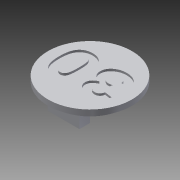
# Autodesk Inventor part: Inside
Saved by Autodesk Inventor 2014 (Build 180170000, 170)
## iProperties
Created: 2017-08-29
Part Number: Inside
Material: Generic
Document SubType Name: Modeling
Designer: resaj
Density: 1 g/cm^3
Appearance: White
Author: resaj
Autodesk Inventor part; units mm, degrees
ref_plane "YZ Plane" through (0, 0, 0) normal (1, 0, 0) x (0, 1, 0)
ref_plane "XZ Plane" through (0, 0, 0) normal (0, 1, 0) x (-1, 0, 0)
sketch "Sketch1" plane through (0, 0, 0) normal (0, 1, 0) x (-1, 0, 0)
  circle A0 centre (0, 0) radius 19.9
  dimension "d0" = 39.8
  constraints: 1 centre point, 1 coincident
  measures "d0" diameter of A0
extrude "Extrusion1" add sketch "Sketch1" along normal blind 2.6
sketch "Sketch2" plane through (0, 0, 0) normal (0, -1, 0) x (1, 0, 0)
  circle A0 centre (0, 0) radius 19.9 projected
  circle A1 centre (0, 0) radius 17.4
  dimension "d3" = 34.8
  constraints: 1 centre point, 1 coincident
  measures "d3" diameter of A1
extrude "Extrusion2" add sketch "Sketch2" along normal blind 2 contours A1
sketch "Sketch3" plane through (0, -2, 0) normal (0, -1, 0) x (1, 0, 0)
  circle A0 centre (0, 0) radius 17.4 projected
  line L0 (0, 0) -> (0, 17.4) construction
  line L1 (0, 0) -> (17.4, 0) construction
  line L2 (0, 12.5) -> (7.5, 12.5)
  line L3 (7.5, 12.5) -> (7.5, 7.5)
  line L4 (7.5, 7.5) -> (0, 7.5)
  line L5 (0, 12.5) -> (-7.5, 12.5)
  line L6 (-7.5, 12.5) -> (-7.5, 7.5)
  line L7 (-7.5, 7.5) -> (0, 7.5)
  line L8 (0, -12.5) -> (7.5, -12.5)
  line L9 (7.5, -12.5) -> (7.5, -7.5)
  line L10 (7.5, -7.5) -> (0, -7.5)
  line L11 (-7.5, -7.5) -> (0, -7.5)
  line L12 (-7.5, -12.5) -> (-7.5, -7.5)
  line L13 (0, -12.5) -> (-7.5, -12.5)
  dimension "d6" = 15
  dimension "d7" = 5
  dimension "d8" = 15
  constraints: 28 end point, 8 symmetric about line, 2 perpendicular, 2 point on circle, 2 point on line, 1 parallel, 1 vertical
  measures "d6" distance between parallel lines of L3 L6
  measures "d7" distance of L2.end L3.end
  measures "d8" distance between parallel lines of L10 L4
extrude "Extrusion3" add sketch "Sketch3" along normal blind 7.5 contours L2 L3 L4 L7 L6 L5 | L13 L12 L11 L10 L9 L8
ref_plane "Work Plane1" through (7.5, -9.5, 10) normal (0, 0, 1) x (1, 0, 0)
sketch "Sketch4" plane through (7.5, -2, -12.5) normal (0, 0, -1) x (-1, 0, 0)
  line L0 (0, 0) -> (15, 0) projected
  line L1 (0, 0) -> (0, -7.5) projected
  line L2 (15, -7.5) -> (0, -7.5) projected
  line L3 (15, 0) -> (15, -7.5) projected
  line L4 (2.35, 0) -> (2.35, -5.15)
  line L5 (2.35, -5.15) -> (12.65, -5.15)
  line L6 (12.65, -5.15) -> (12.65, 0)
  line L7 (2.35, -5.15) -> (0, -5.15) construction
  line L8 (2.35, -5.15) -> (2.35, -7.5) construction
  line L9 (12.65, -5.15) -> (15, -5.15) construction
  point P0 (7.5, 2)
  dimension "d11" = 10.3
  constraints: 12 end point, 7 perpendicular, 5 point on line, 1 parallel
  measures "d11" distance of L4.end L5.end
extrude "Extrusion4" cut sketch "Sketch4" against normal up to surface (22.5 mm away) contours L0 L6 L5 L4
sketch "Sketch5" plane through (0, 2.6, 0) normal (0, 1, 0) x (1, 0, 0)
  line L0 (15.5957, -8.6476) -> (-15.5957, -8.6476) construction
  line L1 (-15.5957, -8.6476) -> (-15.5957, 11.0665) construction
  line L2 (-15.5957, 11.0665) -> (15.5957, 11.0665) construction
  line L3 (15.5957, 11.0665) -> (15.5957, -8.6476) construction
  line L4 (14.5154, 4.6525) -> (10.6853, 4.2456)
  spline S0 degree 2 poles (10.6853, 4.2456) (10.531, 5.5083) (8.8755, 6.8551) (7.7391, 6.8551) knots 0 0 0 1 2 2 2
  spline S1 degree 2 poles (7.7391, 6.8551) (6.5185, 6.8551) (4.8209, 5.2558) (4.8209, 3.8528) knots 0 0 0 1 2 2 2
  spline S2 degree 2 poles (4.8209, 3.8528) (4.8209, 2.548) (6.4483, 1.0469) (7.6128, 1.0469) knots 0 0 0 1 2 2 2
  spline S3 degree 2 poles (7.6128, 1.0469) (8.3704, 1.0469) (9.4226, 1.2994) knots 0 0 0 1 1 1
  line L5 (9.4226, 1.2994) -> (8.9877, -1.5065)
  spline S4 degree 2 poles (8.9877, -1.5065) (7.4444, -1.4785) (6.5465, -2.0958) knots 0 0 0 1 1 1
  spline S5 degree 2 poles (6.5465, -2.0958) (5.6627, -2.7131) (5.6627, -3.8214) knots 0 0 0 1 1 1
  spline S6 degree 2 poles (5.6627, -3.8214) (5.6627, -4.7614) (6.9534, -5.8136) (7.9495, -5.8136) knots 0 0 0 1 2 2 2
  spline S7 degree 2 poles (7.9495, -5.8136) (8.9596, -5.8136) (10.4328, -4.593) (10.573, -3.4005) knots 0 0 0 1 2 2 2
  line L6 (10.573, -3.4005) -> (14.2348, -3.9477)
  spline S8 degree 2 poles (14.2348, -3.9477) (13.6596, -6.4169) (10.3486, -8.6476) (7.8373, -8.6476) knots 0 0 0 1 2 2 2
  spline S9 degree 2 poles (7.8373, -8.6476) (5.0033, -8.6476) (1.6783, -5.7715) (1.6783, -4.0318) knots 0 0 0 1 2 2 2
  spline S10 degree 2 poles (1.6783, -4.0318) (1.6783, -2.8534) (3.1654, -0.9594) (4.6666, -0.2579) knots 0 0 0 1 2 2 2
  spline S11 degree 2 poles (4.6666, -0.2579) (2.9269, 0.0788) (0.7523, 2.3376) (0.7523, 4.0212) knots 0 0 0 1 2 2 2
  spline S12 degree 2 poles (0.7523, 4.0212) (0.7523, 6.4904) (4.863, 9.7172) (7.711, 9.7172) knots 0 0 0 1 2 2 2
  spline S13 degree 2 poles (7.711, 9.7172) (10.4328, 9.7172) (14.2067, 6.9954) (14.5154, 4.6525) knots 0 0 0 1 2 2 2
  spline S14 degree 2 poles (-8.395, -8.6476) (-11.3973, -8.6476) (-15.1152, -4.565) (-15.1152, 0.5418) knots 0 0 0 1 2 2 2
  spline S15 degree 2 poles (-15.1152, 0.5418) (-15.1152, 5.6346) (-11.3973, 9.7172) (-8.409, 9.7172) knots 0 0 0 1 2 2 2
  spline S16 degree 2 poles (-8.409, 9.7172) (-5.4067, 9.7172) (-1.6888, 5.6626) (-1.6888, 0.4997) knots 0 0 0 1 2 2 2
  spline S17 degree 2 poles (-1.6888, 0.4997) (-1.6888, -4.565) (-5.4067, -8.6476) (-8.395, -8.6476) knots 0 0 0 1 2 2 2
  spline S18 degree 2 poles (-8.395, -5.7855) (-7.2165, -5.7855) (-5.8276, -3.5829) (-5.8276, 0.5418) knots 0 0 0 1 2 2 2
  spline S19 degree 2 poles (-5.8276, 0.5418) (-5.8276, 4.6665) (-7.2165, 6.8551) (-8.395, 6.8551) knots 0 0 0 1 2 2 2
  spline S20 degree 2 poles (-8.395, 6.8551) (-9.5735, 6.8551) (-10.9484, 4.6525) (-10.9484, 0.5418) knots 0 0 0 1 2 2 2
  spline S21 degree 2 poles (-10.9484, 0.5418) (-10.9484, -3.5829) (-9.5735, -5.7855) (-8.395, -5.7855) knots 0 0 0 1 2 2 2
  constraints: 2 other
extrude "Extrusion5" cut sketch "Sketch5" against normal blind 1
body "Solid1"
